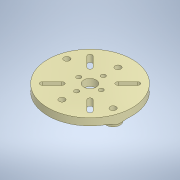
# Autodesk Inventor part: motor_mount
Saved by Autodesk Inventor 2021 (Build 250183000, 183)
## iProperties
Created: 2021-02-03
Part Number: motor_mount
Material: PC/ABS 플라스틱
Document SubType Name: Modeling
Designer: jun85
Density: 0.357273 g/cm^3
Appearance: 매끄러움 - 물푸레나무색
Author: jun85
Autodesk Inventor part; units mm, degrees
ref_plane "YZ Plane" through (0, 0, 0) normal (1, 0, 0) x (0, 1, 0)
ref_plane "XZ Plane" through (0, 0, 0) normal (0, 1, 0) x (-1, 0, 0)
ref_plane "XY Plane" through (0, 0, 0) normal (0, 0, 1) x (1, 0, 0)
sketch "스케치1" plane through (0, 0, 0) normal (0, 1, 0) x (-1, 0, 0)
  line L0 (23.5, -7) -> (-23.5, -7) construction
  line L1 (-23.5, -7) -> (-23.5, 7) construction
  line L2 (-23.5, 7) -> (23.5, 7) construction
  line L3 (23.5, 7) -> (23.5, -7) construction
  circle A0 centre (23.5, -7) radius 2.1
  circle A1 centre (-23.5, 7) radius 2.1
  circle A2 centre (0, -20) radius 2.1
  circle A3 centre (0, 20) radius 2.1
  circle A4 centre (0, 0) radius 4.5
  circle A5 centre (8, 0) radius 1.6
  circle A6 centre (0, 9.5) radius 1.6
  circle A7 centre (-8, 0) radius 1.6
  circle A8 centre (0, -9.5) radius 1.6
  line L4 (8, 0) -> (0, -9.5) construction
  line L5 (0, -9.5) -> (-8, 0) construction
  line L6 (-8, 0) -> (0, 9.5) construction
  line L7 (0, 9.5) -> (8, 0) construction
  line L8 (10, -10) -> (17, -17) construction
  line L9 (8.8686, -11.1314) -> (15.8686, -18.1314)
  line L10 (18.1314, -15.8686) -> (11.1314, -8.8686)
  arc A9 (11.1314, -8.8686) -> (8.8686, -11.1314) centre (10, -10) ccw
  arc A10 (15.8686, -18.1314) -> (18.1314, -15.8686) centre (17, -17) ccw
  line L11 (-10, -10) -> (-17, -17) construction
  line L12 (-11.1314, -8.8686) -> (-18.1314, -15.8686)
  line L13 (-15.8686, -18.1314) -> (-8.8686, -11.1314)
  arc A11 (-8.8686, -11.1314) -> (-11.1314, -8.8686) centre (-10, -10) ccw
  arc A12 (-18.1314, -15.8686) -> (-15.8686, -18.1314) centre (-17, -17) ccw
  line L14 (10, 10) -> (17, 17) construction
  line L15 (11.1314, 8.8686) -> (18.1314, 15.8686)
  line L16 (15.8686, 18.1314) -> (8.8686, 11.1314)
  arc A13 (8.8686, 11.1314) -> (11.1314, 8.8686) centre (10, 10) ccw
  arc A14 (18.1314, 15.8686) -> (15.8686, 18.1314) centre (17, 17) ccw
  line L17 (-10, 10) -> (-17, 17) construction
  line L18 (-8.8686, 11.1314) -> (-15.8686, 18.1314)
  line L19 (-18.1314, 15.8686) -> (-11.1314, 8.8686)
  arc A15 (-11.1314, 8.8686) -> (-8.8686, 11.1314) centre (-10, 10) ccw
  arc A16 (-15.8686, 18.1314) -> (-18.1314, 15.8686) centre (-17, 17) ccw
  line L20 (10, -10) -> (-10, -10) construction
  line L21 (-10, -10) -> (-10, 10) construction
  line L22 (-10, 10) -> (10, 10) construction
  line L23 (10, 10) -> (10, -10) construction
  circle A17 centre (0, 0) radius 30
  line L24 (42, 0) -> (-42, 0) projected
  line L25 (0, -42) -> (0, 42) projected
  line L26 (0, 9.5) -> (0, -9.5) construction
  line L27 (8, 0) -> (-8, 0) construction
  line L28 (28.5, -25) -> (-28.5, -25)
  line L29 (-28.5, -25) -> (-28.5, 25)
  line L30 (-28.5, 25) -> (28.5, 25)
  line L31 (28.5, 25) -> (28.5, -25)
  point P0 (13.5, -13.5)
  point P1 (-13.5, -13.5)
  point P2 (13.5, 13.5)
  point P3 (-13.5, 13.5)
  dimension "d0" = 4.2
  dimension "d1" = 40
  dimension "d2" = 47
  dimension "d3" = 14
  dimension "d4" = 3.2
  dimension "d5" = 16
  dimension "d6" = 19
  dimension "d7" = 9
  dimension "d8" = 20
  dimension "d9" = 34
  dimension "d10" = 1.6
  dimension "d11" = 60
  dimension "d18" = 5
  dimension "d19" = 5
  constraints: 68 end point, 18 centre point, 16 point on circle, 16 tangent, 9 equal radius, 8 parallel, 6 midpoint, 5 coincident, 5 equal length, 5 perpendicular, 3 horizontal, 2 collinear, 1 point on line, 1 vertical, 14 other
  measures "d0" diameter of A2
  measures "d1" distance of A3.centre A2.centre
  measures "d2" distance of L1.end L2.end
  measures "d3" distance of L2.end L0.start
  measures "d4" diameter of A5
  measures "d5" distance of L5.end L4.start
  measures "d6" distance of L6.end L4.end
  measures "d7" diameter of A4
  measures "d8" distance of L8.start L11.start
  measures "d9" distance of L11.end L8.end
  measures "d10" radius of A9
  measures "d11" diameter of A17
  measures "d18" distance from line of L28 A2.centre
  measures "d19" distance from line of L31 A0.centre
extrude "돌출1" add sketch "스케치1" along normal blind 5 contours A2 L25 A8 A4 L24 A5 L31 A17 L28 | A2 L25 L28 A17 L29 L24 A7 A4 A8 | L28 A17 L25 | L25 A17 L28 | L31 L24 A17 | A17 L24 L29 | L24 A7 L29 A17 L30 L25 A3 A6 A4 | A4 L25 A6 A3 L30 A17 L31 L24 A5 | L24 L31 A17 | A17 L29 L24 | L30 L25 A17 | A17 L25 L30
sketch "스케치2" plane through (0, 0, 0) normal (0, -1, 0) x (1, 0, 0)
  circle A0 centre (0, 0) radius 30 projected
  circle A1 centre (0, 0) radius 4.5 projected
  circle A2 centre (8, 0) radius 1.6 projected
  circle A3 centre (0, -20) radius 2.1 projected
  circle A4 centre (0, -9.5) radius 1.6 projected
  circle A5 centre (-8, 0) radius 1.6 projected
  arc A6 (8.8686, 11.1314) -> (11.1314, 8.8686) centre (10, 10) ccw projected
  line L0 (15.8686, 18.1314) -> (8.8686, 11.1314) projected
  arc A7 (18.1314, 15.8686) -> (15.8686, 18.1314) centre (17, 17) ccw projected
  line L1 (11.1314, 8.8686) -> (18.1314, 15.8686) projected
  circle A8 centre (23.5, 7) radius 2.1 projected
  arc A9 (-11.1314, 8.8686) -> (-8.8686, 11.1314) centre (-10, 10) ccw projected
  line L2 (-18.1314, 15.8686) -> (-11.1314, 8.8686) projected
  arc A10 (-15.8686, 18.1314) -> (-18.1314, 15.8686) centre (-17, 17) ccw projected
  line L3 (-8.8686, 11.1314) -> (-15.8686, 18.1314) projected
  circle A11 centre (0, 20) radius 2.1 projected
  circle A12 centre (0, 9.5) radius 1.6 projected
  circle A13 centre (-23.5, -7) radius 2.1 projected
  arc A14 (-8.8686, -11.1314) -> (-11.1314, -8.8686) centre (-10, -10) ccw projected
  line L4 (-15.8686, -18.1314) -> (-8.8686, -11.1314) projected
  arc A15 (-18.1314, -15.8686) -> (-15.8686, -18.1314) centre (-17, -17) ccw projected
  line L5 (-11.1314, -8.8686) -> (-18.1314, -15.8686) projected
  arc A16 (11.1314, -8.8686) -> (8.8686, -11.1314) centre (10, -10) ccw projected
  line L6 (18.1314, -15.8686) -> (11.1314, -8.8686) projected
  arc A17 (15.8686, -18.1314) -> (18.1314, -15.8686) centre (17, -17) ccw projected
  line L7 (8.8686, -11.1314) -> (15.8686, -18.1314) projected
  circle A18 centre (0, 20) radius 5
  circle A19 centre (23.5, 7) radius 2.1 projected
  circle A20 centre (23.5, 7) radius 5
  circle A21 centre (0, -20) radius 2.1 projected
  circle A22 centre (0, -20) radius 5
  circle A23 centre (-23.5, -7) radius 2.1 projected
  circle A24 centre (-23.5, -7) radius 5
  dimension "d14" = 10
  constraints: 4 centre point, 4 coincident, 3 equal radius
  measures "d14" diameter of A20
extrude "돌출2" add sketch "스케치2" along normal blind 3 contours A18 | A20 | A22 | A24
fillet "모깎기1" radius 3 4 edges at (-5, 0, 20) (-28.5, 0, -7) (-5, 0, -20) (18.5, 0, 7)
